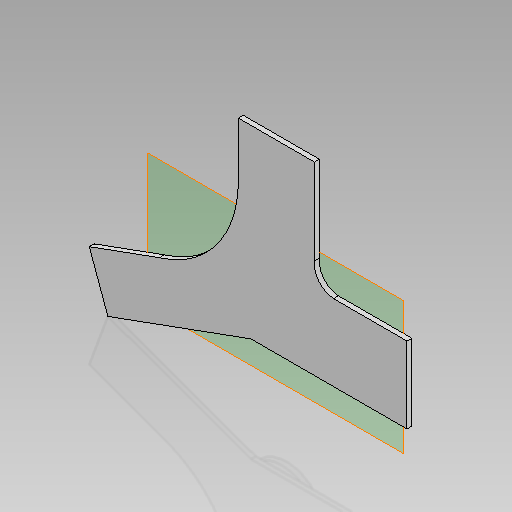
# Autodesk Inventor part: ЛЦМК000002.00.00.00.00.08
Saved by Autodesk Inventor 2021.2 (Build 252289000, 289)
## iProperties
Created: 2025-10-27
Part Number: ЛЦМК000002.00.00.00.00.08
Material: Типовые
Document SubType Name: Modeling
Designer: Захаров
Density: 1 g/cm^3
Appearance: По умолчанию
Author: Захаров
Autodesk Inventor part; units mm, degrees
ref_plane "YZ Plane" through (0, 0, 0) normal (1, 0, 0) x (0, 1, 0)
ref_plane "XZ Plane" through (0, 0, 0) normal (0, 1, 0) x (-1, 0, 0)
ref_plane "XY Plane" through (0, 0, 0) normal (0, 0, 1) x (1, 0, 0)
ref_plane "РабПлоскость1" through (0, 0, -194) normal (0, 0, -1) x (-1, 0, 0)
sketch "Эскиз1" plane through (0, 0, -194) normal (0, 0, -1) x (-1, 0, 0)
  circle A0 centre (0, 0) radius 12
  dimension "d0" = 24
  constraints: 1 centre point, 1 coincident
  measures "d0" diameter of A0
extrude "Выдавливание1" add sketch "Эскиз1" along normal blind 2
sketch "Эскиз2" plane through (0, 0, -196) normal (0, 0, -1) x (-1, 0, 0)
  circle A0 centre (0, 0) radius 14
  dimension "d3" = 28
  constraints: 1 centre point, 1 coincident
  measures "d3" diameter of A0
extrude "Выдавливание2" add sketch "Эскиз2" along normal blind 2
sketch "Эскиз3" plane through (0, 0, -194) normal (0, 0, 1) x (1, 0, 0)
  line L0 (0, -14.0792) -> (7.9343, -14.0792)
  arc A0 (-0.2531, 24.5019) -> (-1.2854, 24.456) centre (0.2785, 0.9208) ccw
  line L1 (0.2785, 0.9208) -> (0.2785, 84.4485) construction
  line L2 (50, 13.9208) -> (23, 13.9208)
  line L3 (0, -14.0792) -> (50, -14.0792)
  line L4 (50, -14.0792) -> (50, 13.9208)
  line L5 (50, 13.9208) -> (0, -14.0792) construction
  line L6 (0, 13.9208) -> (50, -14.0792) construction
  line L7 (16, 53.9208) -> (-12, 53.9208)
  line L8 (16, 22.4208) -> (16, 53.9208)
  line L9 (16, 53.9208) -> (-9.7913, 3.9696) construction
  line L10 (-12, 53.9208) -> (16, -5.6793) construction
  arc A1 (16, 22.4208) -> (23, 13.9208) centre (23.4314, 21.4084) ccw
  line L11 (-7.3772, -14.0792) -> (-60, -33.2323)
  line L12 (-60, -33.2323) -> (-66.8404, -14.4385)
  line L13 (-66.8404, -14.4385) -> (-40.9989, -5.0329)
  line L14 (0, -14.0792) -> (-7.3772, -14.0792)
  arc A2 (-40.9989, -5.0329) -> (-12, 33.9208) centre (-52.4998, 33.7998) ccw
  line L15 (-12, 53.9208) -> (-12, 33.9208)
  arc A3 (1.8425, 24.456) -> (0.8102, 24.5019) centre (0.2785, 0.9208) ccw
  point P0 (0, 0)
  point P1 (0, 13.9208)
  point P2 (-24.4429, -0.0792)
  point P3 (-25, 0)
  point P4 (-0.7823, 25.5269)
  point P5 (0, 0)
  point P6 (25, -0.0792)
  point P7 (25.5571, 0)
  point P8 (1.3394, 25.5269)
  dimension "d21" = 28
  dimension "d22" = 28
  dimension "d23" = 20
  dimension "d24" = 50
  dimension "d25" = 110
  dimension "d26" = 160
  dimension "d27" = 40
  dimension "d28" = 27
  dimension "d29" = 31.5
  dimension "d30" = 20
  dimension "d31" = 27.5
  dimension "d32" = 56
  dimension "d33" = 40.5
  dimension "d34" = 7.5
  dimension "d35" = 34
  dimension "d36" = 53
  dimension "d37" = 50
  constraints: 30 end point, 8 point on circle, 7 point on line, 6 symmetric about line, 4 centre point, 3 parallel, 3 perpendicular, 2 coincident, 2 vertical, 1 horizontal, 1 horizontal alignment, 1 midpoint, 5 other
  measures "d21" distance of L3.end L2.start
  measures "d22" distance of L8.end L10.start
  measures "d23" distance of L11.end L13.start
  measures "d24" distance of L0.start L3.end
  measures "d25" horizontal distance of L3.end L11.end
  measures "d26" angle of L3 L11
  measures "d27" distance from line of L2.start L7
  measures "d28" distance of L2.start L2.end
  measures "d29" distance of L8.start L8.end
  measures "d30" distance of L10.start L15.end
  measures "d31" distance of L13.start L13.end
  measures "d32" distance of L14.end L11.end
  measures "d33" radius of A2
  measures "d34" radius of A1
  measures "d35" distance between parallel lines of L8 L4
  measures "d36" distance from line of L7 L1.start
  measures "d37" distance from line of L4 point (0, 0)
extrude "Выдавливание3" add sketch "Эскиз3" along normal blind 1.8
